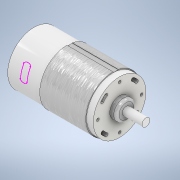
# Autodesk Inventor part: 775motor
Saved by Autodesk Inventor 2020 (Build 240168000, 168)
## iProperties
Created: 2020-03-29
Part Number: 775motor
Material: Generic
Document SubType Name: Modeling
Designer: Manish
Density: 1 g/cm^3
Appearance: Polished Brushed
Author: Manish
Autodesk Inventor part; units mm, degrees
ref_plane "YZ Plane" through (0, 0, 0) normal (1, 0, 0) x (0, 1, 0)
ref_plane "XZ Plane" through (0, 0, 0) normal (0, 1, 0) x (-1, 0, 0)
ref_plane "XY Plane" through (0, 0, 0) normal (0, 0, 1) x (1, 0, 0)
sketch "Sketch1" plane through (0, 0, 0) normal (1, 0, 0) x (0, 1, 0)
  circle A0 centre (0, 0) radius 20
  dimension "d0" = 40
  constraints: 1 centre point, 1 coincident
  measures "d0" diameter of A0
extrude "Extrusion1" add sketch "Sketch1" against normal blind 65
sketch "Sketch2" plane through (0, 0, 0) normal (1, 0, 0) x (0, 0, -1)
  circle A0 centre (0, 0) radius 7.5
  circle A1 centre (0, 0) radius 3
  dimension "d3" = 15
  dimension "d4" = 6
  constraints: 2 centre point, 2 coincident
  measures "d3" diameter of A0
  measures "d4" diameter of A1
extrude "Extrusion2" add sketch "Sketch2" along normal blind 5
fillet "Fillet1" radius 2 1 edges at (5, 0, 7.5)
sketch "Sketch3" plane through (0, 0, 0) normal (1, 0, 0) x (0, 0, -1)
  circle A0 centre (0, 0) radius 20.7096
  circle A1 centre (0, 0) radius 20.0622
  constraints: 2 centre point, 2 coincident
extrude "Extrusion3" add sketch "Sketch3" against normal blind 40
sketch "Sketch4" plane through (0, 0, 0) normal (1, 0, 0) x (0, 0, -1)
  circle A0 centre (0, 0) radius 20.0395
  circle A1 centre (0, 0) radius 20.0395
  circle A2 centre (0, 0) radius 20.7096
  constraints: 3 centre point, 3 coincident, 1 concentric
extrude "Extrusion4" cut sketch "Sketch4" against normal blind 5
sketch "Sketch5" plane through (-5, 0, 0) normal (1, 0, 0) x (0, 0, -1)
  circle A0 centre (0, 0) radius 20.0622 projected
  circle A1 centre (0, 0) radius 20.7096 projected
  line L0 (0, 20.0622) -> (0, 20.7096)
  line L1 (0, 20.7096) -> (4, 20.7096)
  line L2 (4, 20.7096) -> (4, 20.0622)
  line L3 (4, 20.0622) -> (0, 20.0622)
  dimension "d12" = 4
  constraints: 8 end point, 2 parallel, 2 vertical alignment, 1 perpendicular, 1 vertical, 2 other
  measures "d12" distance of L0.end L1.end
extrude "Extrusion5" cut sketch "Sketch5" against normal through all contours L0 A1 L2 L3 | L1 L2 A1 picked at (2.2253, 20.2201)
sketch "Sketch6" plane through (0, 0, 0) normal (1, 0, 0) x (0, 0, -1)
  circle A0 centre (0, 0) radius 17.7894
  circle A1 centre (0, 0) radius 15.3585
  arc A2 (-10.7216, -14.1954) -> (-9.2565, -12.2556) centre (-9.989, -13.2255) ccw
  arc A3 (-11.811, -9.8174) -> (-13.9091, -11.0905) centre (-12.9418, -10.3192) ccw
  arc A4 (-14.1954, 10.7216) -> (-12.2556, 9.2565) centre (-13.2255, 9.989) ccw
  arc A5 (-9.8174, 11.811) -> (-11.0905, 13.9091) centre (-10.3192, 12.9418) ccw
  arc A6 (10.7216, 14.1954) -> (9.2565, 12.2556) centre (9.989, 13.2255) ccw
  arc A7 (11.811, 9.8174) -> (13.9091, 11.0905) centre (12.9418, 10.3192) ccw
  arc A8 (14.1954, -10.7216) -> (12.2556, -9.2565) centre (13.2255, -9.989) ccw
  arc A9 (9.8174, -11.811) -> (11.0905, -13.9091) centre (10.3192, -12.9418) ccw
  circle A10 centre (0, -16.5738) radius 1.0703
  circle A11 centre (16.5738, 0) radius 1.0703
  circle A12 centre (0, 16.5738) radius 1.0703
  circle A13 centre (-16.5738, 0) radius 1.0703
  point P0 (9.3285, -12.2009)
  point P1 (14.1954, -10.7216)
  point P2 (12.2556, -9.2565)
  point P3 (12.2009, 9.3285)
  point P4 (10.7216, 14.1954)
  point P5 (9.2565, 12.2556)
  point P6 (-9.3285, 12.2009)
  point P7 (-11.0905, 13.9091)
  point P8 (-14.1954, 10.7216)
  point P9 (-12.2009, -9.3285)
  dimension "d17" = 360
  dimension "d21" = 360
  constraints: 20 point on circle, 14 centre point, 2 coincident, 2 tangent, 46 other
extrude "Extrusion6" cut sketch "Sketch6" against normal blind 10 contours A7 A1 A6 A0 | A0 A9 A1 A8 | A5 A1 A4 A0 | A0 A3 A1 A2 | A10 | A11 | A12 | A13
sketch3d "3D Sketch1"
sketch "Sketch8" plane through (-65, 0, 0) normal (-1, 0, 0) x (0, 0, 1)
  circle A0 centre (0, 0) radius 18.7114
  circle A1 centre (0, 0) radius 7.5 projected
  circle A2 centre (0, 0) radius 5
  constraints: 2 centre point, 2 coincident
extrude "Extrusion7" cut sketch "Sketch8" against normal blind 2 contours A0
sketch "Sketch9" plane through (0, 0, 0) normal (1, 0, 0) x (0, 0, -1)
  circle A0 centre (0, 0) radius 3 projected
  circle A1 centre (0, 0) radius 5
  circle A2 centre (0, 0) radius 3
  constraints: 2 centre point, 2 coincident, 1 concentric
extrude "Extrusion8" add sketch "Sketch9" along normal blind 20 contours A0
body "Solid1"
